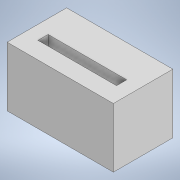
# Autodesk Inventor part: ServoOverServo
Saved by Autodesk Inventor 2020.1 (Build 241239000, 239)
## iProperties
Created: 2020-06-07
Part Number: ServoOverServo
Material: Generic
Document SubType Name: Modeling
Designer: super
Density: 1 g/cm^3
Appearance: Default
Author: super
Autodesk Inventor part; units mm, degrees
ref_plane "YZ Plane" through (0, 0, 0) normal (1, 0, 0) x (0, 1, 0)
ref_plane "XZ Plane" through (0, 0, 0) normal (0, 1, 0) x (-1, 0, 0)
ref_plane "XY Plane" through (0, 0, 0) normal (0, 0, 1) x (1, 0, 0)
sketch "Sketch1" plane through (0, 0, 0) normal (0, 1, 0) x (-1, 0, 0)
  line L0 (0, 0) -> (-25, 0)
  line L1 (-25, 0) -> (-25, -14)
  line L2 (-25, -14) -> (0, -14)
  line L3 (0, -14) -> (0, 0)
  dimension "d0" = 25
  dimension "d1" = 14
  constraints: 8 end point, 2 parallel, 1 horizontal, 1 perpendicular
  measures "d0" distance of L2.end L1.end
  measures "d1" distance of L1.end L0.end
extrude "Extrusion1" add sketch "Sketch1" along normal blind 14
sketch "Sketch2" plane through (0, 14, 0) normal (0, 1, 0) x (1, 0, 0)
  line L0 (3.25, 4) -> (21.75, 4)
  line L1 (21.75, 4) -> (21.75, 6.4)
  line L2 (21.75, 6.4) -> (3.25, 6.4)
  line L3 (3.25, 6.4) -> (3.25, 4)
  point P0 (0, 0)
  dimension "d6" = 18.5
  dimension "d7" = 2.4
  constraints: 8 end point, 3 perpendicular, 1 horizontal
  measures "d6" distance of L0.start L0.end
  measures "d7" distance of L0.end L1.end
extrude "Extrusion2" cut sketch "Sketch2" against normal blind 10.3
body "Solid1"
